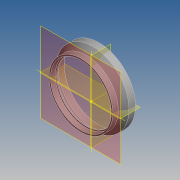
# Autodesk Inventor part: P012_Canon_AdaptCoudeTube
Saved by Autodesk Inventor 2020 (Build 240168000, 168)
## iProperties
Created: 2021-10-21
Part Number: P012_Canon_AdaptCoudeTube
Material: Générique
Document SubType Name: Modeling
Designer: gabri
Density: 1 g/cm^3
Appearance: Par défaut
Author: gabri
Autodesk Inventor part; units mm, degrees
sketch "Esquisse2" plane through (0, 0, 0) normal (0, 0, 1) x (1, 0, 0)
  line L0 (-8.75, 36.8757) -> (-8.75, -38.6317)
  line L1 (20, 15) -> (20, 10)
  line L2 (16.25, 4) -> (16.25, 0)
  line L3 (20, 10) -> (16.25, 5)
  line L4 (16.25, 0) -> (17.45, 0)
  line L5 (17.45, 0) -> (17.45, 4.6)
  line L6 (17.45, 4.6) -> (21.2, 9.6)
  line L7 (21.2, 9.6) -> (21.2, 15)
  line L8 (21.2, 15) -> (20, 15)
  line L9 (16.25, 5) -> (15.25, 5)
  line L10 (15.25, 5) -> (15.25, 4)
  line L11 (15.25, 4) -> (16.25, 4)
  line L12 (-14.74, 0) -> (27.19, 0) construction
  line L13 (0, 51.9772) -> (0, -53.7332) construction
  point P0 (0, 0)
  dimension "d0" = 57.5
  dimension "d1" = 50
  dimension "d3" = 5
  dimension "d4" = 5
  dimension "d5" = 5
  dimension "d6" = 1.2
  dimension "d7" = 1.2
  dimension "d8" = 1.2
  dimension "d10" = 1
  dimension "d11" = 1
  dimension "d12" = 143.13
  dimension "d13" = 5
  dimension "d14" = 4.6
  dimension "d15" = 5.4
  dimension "d16" = 0
  dimension "d17" = 20
  constraints: 24 end point, 4 perpendicular, 3 vertical, 2 horizontal, 2 parallel, 1 other
  measures "d0" diameter of L1 L0
  measures "d1" diameter of L2 L0
  measures "d3" distance of L3.end L2.end
  measures "d4" distance of L1.start L1.end
  measures "d5" vertical distance of L1.end L3.end
  measures "d6" distance between parallel lines of L5 L2
  measures "d7" distance between parallel lines of L6 L3
  measures "d8" distance between parallel lines of L7 L1
  measures "d10" distance of L9.end L10.end
  measures "d11" distance between parallel lines of L2 L10
  measures "d12" angle of L3 L1
  measures "d13" vertical distance of L5.end L6.end
  measures "d14" distance of L4.end L5.end
  measures "d15" distance of L6.end L7.end
  measures "d16" distance between parallel lines of L12 L4
  measures "d17" distance of the line from the sketch origin of L1
revolve "Révolution1" add sketch "Esquisse2" angle 360 about axis through (-8.75, 36.8757, 0) along (0, -1, 0)
